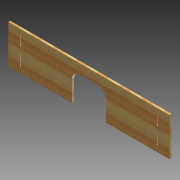
# Autodesk Inventor part: plywood front pannel
Saved by Autodesk Inventor 2012 (Build 160160000, 160)
## iProperties
Created: 2013-09-02
Part Number: plywood front pannel
Material: Default
Document SubType Name: Modeling
Designer: Bryce
Density: 1 g/cm^3
Author: Bryce
Autodesk Inventor part; units mm, degrees
ref_plane "YZ Plane" through (0, 0, 0) normal (1, 0, 0) x (0, 1, 0)
ref_plane "XZ Plane" through (0, 0, 0) normal (0, 1, 0) x (-1, 0, 0)
ref_plane "XY Plane" through (0, 0, 0) normal (0, 0, 1) x (1, 0, 0)
sketch "Sketch1" plane through (0, 0, 0) normal (0, 0, 1) x (1, 0, 0)
  line L0 (965.2, 0) -> (965.2, 228.6)
  line L1 (965.2, 228.6) -> (0, 228.6)
  line L2 (0, 228.6) -> (0, 0)
  line L3 (584.2, 0) -> (584.2, 120.65)
  line L4 (584.2, 171.45) -> (533.4, 171.45) construction
  line L5 (381, 171.45) -> (381, 120.65) construction
  line L6 (0, 0) -> (381, 0)
  line L7 (584.2, 0) -> (965.2, 0)
  arc A0 (431.8, 171.45) -> (381, 120.65) centre (431.8, 120.65) ccw
  arc A1 (584.2, 120.65) -> (533.4, 171.45) centre (533.4, 120.65) ccw
  line L8 (431.8, 171.45) -> (381, 171.45) construction
  line L9 (381, 120.65) -> (381, 0)
  line L10 (533.4, 171.45) -> (431.8, 171.45)
  line L11 (584.2, 120.65) -> (584.2, 171.45) construction
  line L12 (69.85, 201.93) -> (76.2, 201.93)
  line L13 (76.2, 201.93) -> (76.2, 138.43)
  line L14 (76.2, 138.43) -> (69.85, 138.43)
  line L15 (69.85, 138.43) -> (69.85, 201.93)
  line L16 (69.85, 100.33) -> (76.2, 100.33)
  line L17 (76.2, 100.33) -> (76.2, 36.83)
  line L18 (76.2, 36.83) -> (69.85, 36.83)
  line L19 (69.85, 36.83) -> (69.85, 100.33)
  line L20 (895.35, 201.93) -> (889, 201.93)
  line L21 (889, 201.93) -> (889, 138.43)
  line L22 (889, 138.43) -> (895.35, 138.43)
  line L23 (895.35, 138.43) -> (895.35, 201.93)
  line L24 (895.35, 100.33) -> (889, 100.33)
  line L25 (889, 100.33) -> (889, 36.83)
  line L26 (889, 36.83) -> (895.35, 36.83)
  line L27 (895.35, 36.83) -> (895.35, 100.33)
  dimension "d0" = 965.2
  dimension "d1" = 228.6
  dimension "d4" = 203.2
  dimension "d6" = 381
  dimension "d7" = 171.45
  dimension "d8" = 50.8
  dimension "d9" = 69.85
  dimension "d10" = 6.35
  dimension "d11" = 63.5
  dimension "d12" = 63.5
  dimension "d13" = 101.6
  dimension "d14" = 26.67
  dimension "d15" = 6.35
  dimension "d16" = 69.85
  dimension "d17" = 63.5
  dimension "d18" = 63.5
  dimension "d19" = 101.6
  dimension "d20" = 26.67
  constraints: 56 end point, 17 parallel, 12 perpendicular, 10 tangent, 6 horizontal, 4 point on circle, 3 collinear, 2 centre point, 1 equal radius
  measures "d0" distance of L0.end L1.end
  measures "d1" distance of L1.end L2.end
  measures "d4" distance of L4.start L5.start
  measures "d6" distance between parallel lines of L2 L5
  measures "d7" distance of L5.start L6.end
  measures "d8" radius of A0
  measures "d9" distance between parallel lines of L2 L15
  measures "d10" distance of L12.start L12.end
  measures "d11" distance of L14.end L12.start
  measures "d12" distance of L18.end L16.start
  measures "d13" distance between parallel lines of L18 L14
  measures "d14" distance between parallel lines of L1 L12
  measures "d15" distance of L20.start L20.end
  measures "d16" distance between parallel lines of L0 L23
  measures "d17" distance of L22.end L20.start
  measures "d18" distance of L26.end L24.start
  measures "d19" distance between parallel lines of L26 L22
  measures "d20" distance between parallel lines of L1 L20
extrude "Extrusion1" add sketch "Sketch1" along normal blind 12.7
equation "\"d6\" = 0.5 * d0 - 0.5 * d4"
equation "\"d12\" = d11"
equation "\"d18\" = d17"
equation "\"d20\" = d14"
body "Solid1"
